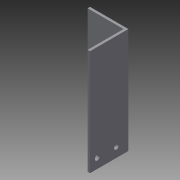
# Autodesk Inventor part: 2x2 angle vertical right
Saved by Autodesk Inventor 2015 SP1 (Build 190203100, 203)
## iProperties
Created: 2015-01-16
Part Number: 2x2 angle vertical right
Material: Generic
Document SubType Name: Modeling
Designer: Jarod
Density: 1 g/cm^3
Appearance: Default
Author: Jarod
Autodesk Inventor part; units mm, degrees
ref_plane "YZ Plane" through (0, 0, 0) normal (1, 0, 0) x (0, 1, 0)
ref_plane "XZ Plane" through (0, 0, 0) normal (0, 1, 0) x (-1, 0, 0)
ref_plane "XY Plane" through (0, 0, 0) normal (0, 0, 1) x (1, 0, 0)
sketch "Sketch1" plane through (0, 0, 0) normal (0, 1, 0) x (-1, 0, 0)
  line L0 (0, 0) -> (3.175, 0)
  line L1 (3.175, 0) -> (3.175, 50.8)
  line L2 (3.175, 50.8) -> (0, 50.8)
  line L3 (0, 50.8) -> (0, 0)
  line L4 (0, 0) -> (50.8, 0)
  line L5 (50.8, 0) -> (50.8, 3.175)
  line L6 (50.8, 3.175) -> (0, 3.175)
  line L7 (0, 3.175) -> (0, 0)
  dimension "d0" = 3.175
  dimension "d1" = 50.8
  dimension "d2" = 50.8
  dimension "d3" = 3.175
  constraints: 16 end point, 4 parallel, 2 horizontal, 2 perpendicular
  measures "d0" distance of L2.end L1.end
  measures "d1" distance of L1.end L0.end
  measures "d2" distance of L6.end L5.end
  measures "d3" distance of L5.end L4.end
extrude "Extrusion1" add sketch "Sketch1" against normal blind 139.7
sketch "Sketch3" plane through (0, 0, 50.8) normal (1, 0, 0) x (0, 0, -1)
  line L0 (50.8, -139.7) -> (0, -139.7) projected
  line L1 (50.8, 0) -> (50.8, -139.7) projected
  line L2 (0, 0) -> (50.8, 0) projected
  line L3 (0, 0) -> (0, -139.7) projected
  point P0 (9.525, -127)
  point P1 (34.925, -127)
  dimension "d17" = 12.7
  dimension "d18" = 9.525
  dimension "d19" = 15.875
  dimension "d20" = 12.7
  measures "d17" distance from line of L0 point (9.525, -127)
  measures "d18" distance from line of L3 point (9.525, -127)
  measures "d19" distance from line of L1 point (34.925, -127)
  measures "d20" distance from line of L0 point (34.925, -127)
hole "Hole2" at (0, -127, 41.275) at (0, -127, 15.875) direction (-1, 0, 0) diameter 6.35 end through all
sketch "Sketch4" plane through (0, 0, 0) normal (0, 0, -1) x (-1, 0, 0)
  line L0 (0, 0) -> (50.8, 0) projected
  line L1 (0, 0) -> (0, -139.7) projected
  line L2 (50.8, -139.7) -> (0, -139.7) projected
  line L3 (50.8, 0) -> (50.8, -139.7) projected
  point P0 (28.575, -63.5)
  point P1 (28.575, -101.6)
  dimension "d28" = 28.575
  dimension "d29" = 63.5
  dimension "d30" = 101.6
  dimension "d31" = 28.575
  measures "d28" distance from line of L1 point (28.575, -63.5)
  measures "d29" distance from line of point (28.575, -63.5) L0
  measures "d30" distance from line of L0 point (28.575, -101.6)
  measures "d31" distance from line of L1 point (28.575, -101.6)
hole "Hole3" at (-28.575, -63.5, 0) at (-28.575, -101.6, 0) direction (0, 0, 1) diameter 6.35 end through all
sketch "Sketch5" plane through (0, 0, 0) normal (0, 1, 0) x (1, 0, 0)
  line L0 (0, 0) -> (-3.175, 0)
  line L1 (-3.175, 0) -> (-3.175, -50.8)
  line L2 (-3.175, -50.8) -> (0, -50.8)
  line L3 (0, -50.8) -> (0, 0)
  constraints: 8 end point, 2 parallel, 1 horizontal, 1 perpendicular
extrude "Extrusion2" add sketch "Sketch5" along normal blind 50.8
sketch "Sketch6" plane through (0, -139.7, 50.8) normal (1, 0, 0) x (0, 0, -1)
  circle A0 centre (9.525, 12.7) radius 3.175 projected
  circle A1 centre (34.925, 12.7) radius 3.175 projected
  line L0 (0, 0) -> (0, 190.5) projected
  line L1 (50.8, 0) -> (0, 0) projected
  line L2 (50.8, 190.5) -> (50.8, 0) projected
  line L3 (0, 190.5) -> (50.8, 190.5) projected
  point P0 (50.8, 139.7)
  point P1 (12.7, 152.4)
  point P2 (38.1, 152.4)
  point P3 (12.7, 177.8)
  point P4 (38.1, 177.8)
  dimension "d41" = 38.1
  dimension "d42" = 12.7
  dimension "d43" = 12.7
  dimension "d44" = 38.1
  dimension "d45" = 12.7
  dimension "d46" = 12.7
  dimension "d47" = 12.7
  dimension "d48" = 12.7
  measures "d41" distance from line of L3 point (12.7, 152.4)
  measures "d42" distance from line of L0 point (12.7, 152.4)
  measures "d43" distance from line of L2 point (38.1, 152.4)
  measures "d44" distance from line of L3 point (38.1, 152.4)
  measures "d45" distance from line of L3 point (12.7, 177.8)
  measures "d46" distance from line of L3 point (38.1, 177.8)
  measures "d47" distance from line of L2 point (38.1, 177.8)
  measures "d48" distance from line of L0 point (12.7, 177.8)
hole "Hole4" at (0, 12.7, 38.1) at (0, 12.7, 12.7) at (0, 38.1, 38.1) at (0, 38.1, 12.7) direction (-1, 0, 0) diameter 6.35 end through all
body "Solid1"
